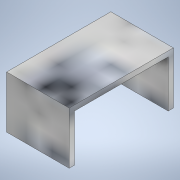
# Autodesk Inventor part: Table
Saved by Autodesk Inventor 2022 (Build 260153000, 153)
## iProperties
Created: 2021-11-27
Part Number: Table
Material: PC/ABS Plastic
Document SubType Name: Modeling
Designer: John Doe
Mass: 0.333715 g
Surface Area: 16.3225 cm^2
Volume: 0.934063 cm^3
Density: 0.357273 g/cm^3
Appearance: Split-Face Stacked - Gray
Author: John Doe
Autodesk Inventor part; units mm, degrees
ref_plane "YZ Plane" through (0, 0, 0) normal (1, 0, 0) x (0, 1, 0)
ref_plane "XZ Plane" through (0, 0, 0) normal (0, 1, 0) x (-1, 0, 0)
ref_plane "XY Plane" through (0, 0, 0) normal (0, 0, 1) x (1, 0, 0)
sketch "Sketch1" plane through (0, 0, 0) normal (1, 0, 0) x (0, 1, 0)
  line L0 (0, 0) -> (12.7, 0)
  line L1 (12.7, 0) -> (12.7, -25.4)
  line L2 (12.7, -25.4) -> (0, -25.4)
  line L3 (0, -25.4) -> (0, -24.13)
  line L4 (0, -24.13) -> (11.43, -24.13)
  line L5 (11.43, -24.13) -> (11.43, -1.27)
  line L6 (11.43, -1.27) -> (0, -1.27)
  line L7 (0, -1.27) -> (0, 0)
  line L8 (5.715, 0) -> (5.715, -1.27) construction
  line L9 (12.7, -12.7) -> (11.43, -12.7) construction
  line L10 (6.35, -25.4) -> (6.35, -24.13) construction
  dimension "d0" = 25.4
  dimension "d1" = 1.27
  dimension "d2" = 12.7
  constraints: 22 end point, 9 perpendicular, 4 midpoint, 3 point on line, 2 equal length, 1 horizontal, 1 parallel
  measures "d0" distance between parallel lines of L2 L0
  measures "d1" distance of L8.start L8.end
  measures "d2" distance between parallel lines of L3 L1
extrude "Extrusion1" add sketch "Sketch1" along normal blind 15.24
body "Solid1"
